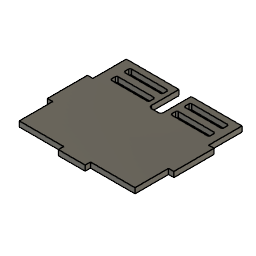
Muur Klein (Autodesk Fusion 360 design; units mm, degrees)
part number: 2026-03-19-13-37-28-850
Autodesk Fusion 360 part; units mm, degrees
note: some values were not read from the file. Set by a fixed rule: which sketch regions a step uses.
sketch "Sketch1" plane through (0, 0, 0) normal (0, 0, 1) x (1, 0, 0)
  line L0 (15.3385, -44.7871) -> (15.3385, -48.7871)
  line L1 (15.3385, -48.7871) -> (-4.6615, -48.7871)
  line L2 (-4.6615, -48.7871) -> (-4.6615, -44.7871)
  line L3 (-37.9015, -44.7871) -> (-4.6615, -44.7871)
  line L4 (15.3385, -44.7871) -> (48.5785, -44.7871)
  line L5 (-37.9015, -19.7871) -> (-41.9015, -19.7871)
  line L6 (-41.9015, -19.7871) -> (-41.9015, 10.2129)
  line L7 (-41.9015, 10.2129) -> (-37.9015, 10.2129)
  line L8 (-37.9015, -19.7871) -> (-37.9015, -44.7871)
  line L9 (-37.9015, 10.2129) -> (-37.9015, 35.2129)
  line L10 (48.5785, 10.2129) -> (52.5785, 10.2129)
  line L11 (52.5785, 10.2129) -> (52.5785, -19.7871)
  line L12 (52.5785, -19.7871) -> (48.5785, -19.7871)
  line L13 (48.5785, -19.7871) -> (48.5785, -21.9637)
  line L14 (48.5785, -21.9637) -> (48.5785, -44.7871)
  line L15 (48.5785, 10.2129) -> (48.5785, 13.5404)
  line L16 (48.5785, 13.5404) -> (48.5785, 35.2129)
  line L17 (-29.5277, 30.6619) -> (-2.944, 30.6619)
  line L18 (-1.944, 29.6619) -> (-1.944, 26.8722)
  line L19 (-2.944, 25.8722) -> (-29.5277, 25.8722)
  line L20 (-30.5277, 26.8722) -> (-30.5277, 29.6619)
  arc A0 (-30.5277, 26.8722) -> (-29.5277, 25.8722) centre (-29.5277, 26.8722) ccw
  arc A1 (-29.5277, 30.6619) -> (-30.5277, 29.6619) centre (-29.5277, 29.6619) ccw
  arc A2 (-1.944, 29.6619) -> (-2.944, 30.6619) centre (-2.944, 29.6619) ccw
  arc A3 (-2.944, 25.8722) -> (-1.944, 26.8722) centre (-2.944, 26.8722) ccw
  line L21 (-30.5277, 16.8722) -> (-30.5277, 19.6619)
  line L22 (-29.5277, 20.6619) -> (-2.944, 20.6619)
  arc A4 (-1.944, 19.6619) -> (-2.944, 20.6619) centre (-2.944, 19.6619) ccw
  line L23 (-1.944, 19.6619) -> (-1.944, 16.8722)
  arc A5 (-29.5277, 20.6619) -> (-30.5277, 19.6619) centre (-29.5277, 19.6619) ccw
  arc A6 (-2.944, 15.8722) -> (-1.944, 16.8722) centre (-2.944, 16.8722) ccw
  arc A7 (-30.5277, 16.8722) -> (-29.5277, 15.8722) centre (-29.5277, 16.8722) ccw
  line L24 (-2.944, 15.8722) -> (-29.5277, 15.8722)
  arc A8 (42.056, 25.8722) -> (43.056, 26.8722) centre (42.056, 26.8722) ccw
  line L25 (42.056, 25.8722) -> (15.4723, 25.8722)
  line L26 (14.4723, 26.8722) -> (14.4723, 29.6619)
  arc A9 (14.4723, 16.8722) -> (15.4723, 15.8722) centre (15.4723, 16.8722) ccw
  arc A10 (15.4723, 20.6619) -> (14.4723, 19.6619) centre (15.4723, 19.6619) ccw
  arc A11 (42.056, 15.8722) -> (43.056, 16.8722) centre (42.056, 16.8722) ccw
  arc A12 (43.056, 19.6619) -> (42.056, 20.6619) centre (42.056, 19.6619) ccw
  arc A13 (15.4723, 30.6619) -> (14.4723, 29.6619) centre (15.4723, 29.6619) ccw
  line L27 (42.056, 15.8722) -> (15.4723, 15.8722)
  line L28 (43.056, 29.6619) -> (43.056, 26.8722)
  arc A14 (14.4723, 26.8722) -> (15.4723, 25.8722) centre (15.4723, 26.8722) ccw
  line L29 (43.056, 19.6619) -> (43.056, 16.8722)
  line L30 (15.4723, 30.6619) -> (42.056, 30.6619)
  line L31 (14.4723, 16.8722) -> (14.4723, 19.6619)
  line L32 (15.4723, 20.6619) -> (42.056, 20.6619)
  arc A15 (43.056, 29.6619) -> (42.056, 30.6619) centre (42.056, 29.6619) ccw
  line L33 (10.5491, 35.2129) -> (10.5491, 14.5299)
  line L34 (8.5491, 12.5299) -> (3.4812, 12.5299)
  line L35 (1.4812, 14.5299) -> (1.4812, 35.2129)
  arc A16 (1.4812, 14.5299) -> (3.4812, 12.5299) centre (3.4812, 14.5299) ccw
  arc A17 (8.5491, 12.5299) -> (10.5491, 14.5299) centre (8.5491, 14.5299) ccw
  line L36 (10.5491, 35.2129) -> (48.5785, 35.2129)
  line L37 (1.4812, 35.2129) -> (-37.9015, 35.2129)
  constraint vertical L0
  constraint horizontal L1
  constraint vertical L2
  constraint perpendicular L2 L3
  constraint horizontal L5
  constraint vertical L6
  constraint horizontal L7
  constraint perpendicular L3 L8
  constraint horizontal L10
  constraint vertical L11
  constraint horizontal L12
  constraint perpendicular L4 L14
  constraint horizontal L17
  constraint vertical L18
  constraint horizontal L19
  constraint vertical L20
  constraint tangent L19 A0
  constraint tangent L20 A0
  constraint tangent L17 A1
  constraint tangent L20 A1
  constraint equal A0 A1
  constraint tangent L17 A2
  constraint tangent L18 A2
  constraint equal A0 A2
  constraint tangent L18 A3
  constraint tangent L19 A3
  constraint equal A0 A3
  constraint horizontal L22
  constraint vertical L23
  constraint horizontal L24
  constraint vertical L21
  constraint tangent A7 L24
  constraint tangent L21 A7
  constraint tangent L22 A5
  constraint tangent L21 A5
  constraint equal A5 A7
  constraint tangent L22 A4
  constraint tangent A4 L23
  constraint equal A4 A7
  constraint tangent L23 A6
  constraint tangent A6 L24
  constraint equal A6 A7
  constraint horizontal L30
  constraint vertical L28
  constraint horizontal L25
  constraint vertical L26
  constraint tangent L25 A14
  constraint tangent L26 A14
  constraint tangent A13 L30
  constraint tangent L26 A13
  constraint equal A13 A14
  constraint tangent L30 A15
  constraint tangent L28 A15
  constraint equal A14 A15
  constraint tangent A8 L28
  constraint tangent A8 L25
  constraint equal A8 A14
  constraint horizontal L32
  constraint vertical L29
  constraint horizontal L27
  constraint vertical L31
  constraint tangent A9 L27
  constraint tangent A9 L31
  constraint tangent A10 L32
  constraint tangent A10 L31
  constraint equal A9 A10
  constraint tangent A12 L32
  constraint tangent A12 L29
  constraint equal A9 A12
  constraint tangent A11 L29
  constraint tangent A11 L27
  constraint equal A9 A11
  constraint vertical L33
  constraint horizontal L34
  constraint vertical L35
  constraint tangent L34 A16
  constraint tangent L35 A16
  constraint tangent L33 A17
  constraint tangent L34 A17
  constraint perpendicular L16 L36
  constraint perpendicular L35 L37
extrude "Extrude1" add sketch "Sketch1" along normal blind 4
